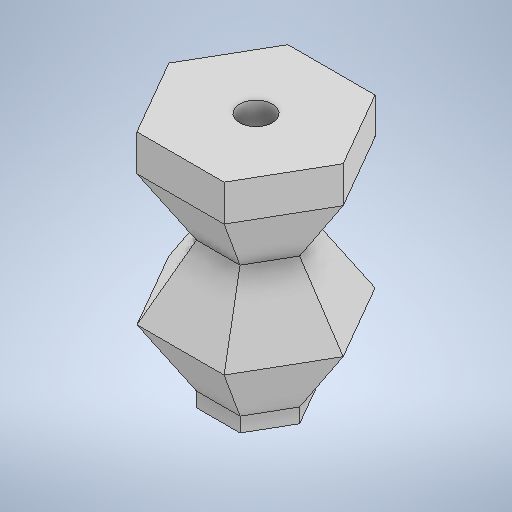
# Autodesk Inventor part: n_6
Saved by Autodesk Inventor 2025.1 (Build 291241000, 241)
## iProperties
Created: 2024-08-13
Part Number: n_6
Material: 일반
Document SubType Name: Modeling
Designer: 82103
Density: 1 g/cm^3
Appearance: 기본값
Author: 82103
Autodesk Inventor part; units mm, degrees
ref_plane "YZ Plane" through (0, 0, 0) normal (1, 0, 0) x (0, 1, 0)
ref_plane "XY Plane" through (0, 0, 0) normal (0, 0, 1) x (1, 0, 0)
sketch "스케치1" plane through (0, 0, 0) normal (0, 1, 0) x (-1, 0, 0)
  line L0 (12, 0) -> (6, -10.3923)
  line L1 (6, -10.3923) -> (-6, -10.3923)
  line L2 (-6, -10.3923) -> (-12, 0)
  line L3 (-12, 0) -> (-6, 10.3923)
  line L4 (-6, 10.3923) -> (6, 10.3923)
  line L5 (6, 10.3923) -> (12, 0)
  point P0 (0, 0)
  point P1 (0, 0)
  dimension "d0" = 24
  constraints: 12 end point, 1 coincident, 1 horizontal alignment, 13 other
  measures "d0" distance of L2.end L0.start
ref_plane "작업 평면1" through (0, 9, 0) normal (0, 1, 0) x (-1, 0, 0)
sketch "스케치2" plane through (0, 9, 0) normal (0, 1, 0) x (-1, 0, 0)
  line L0 (3, -5.1962) -> (-3, -5.1962)
  line L1 (-3, -5.1962) -> (-6, 0)
  line L2 (-6, 0) -> (-3, 5.1962)
  line L3 (-3, 5.1962) -> (3, 5.1962)
  line L4 (3, 5.1962) -> (6, 0)
  line L5 (6, 0) -> (3, -5.1962)
  point P0 (0, 0)
  point P1 (0, 0)
  dimension "d2" = 12
  constraints: 12 end point, 1 coincident, 1 horizontal alignment, 13 other
  measures "d2" distance of L1.end L4.end
loft "로프트1" add profiles "스케치2", "스케치1"
mirror "미러1" about plane through (0, 9, 0) normal (0, 1, 0) of "로프트1"
ref_plane "작업 평면2" through (0, 0, 0) normal (0, 1, 0) x (-1, 0, 0)
mirror "미러2" about plane through (0, 0, 0) normal (0, 1, 0) of "로프트1"
shell "쉘1" thickness 0.5 removed faces 0 ; own thickness 2 on faces at (-8.25, -1.5, 4.7631) (0, -1.5, 9.5263) (8.25, -1.5, 4.7631) (8.25, -1.5, -4.7631) (0, -1.5, -9.5263) (-8.25, -1.5, -4.7631) (-8.25, 16.5, -4.7631) (-8.25, 16.5, 4.7631) (0, 16.5, 9.5263) (8.25, 16.5, 4.7631) (8.25, 16.5, -4.7631) (0, 16.5, -9.5263)
sketch "스케치3" plane through (-3, -9, -5.1962) normal (0, -1, 0) x (1, 0, 0)
  line L0 (0, 0) -> (6, 0) projected
  line L1 (6, 0) -> (9, 5.1962) projected
  line L2 (9, 5.1962) -> (6, 10.3923) projected
  line L3 (6, 10.3923) -> (0, 10.3923) projected
  line L4 (0, 10.3923) -> (-3, 5.1962) projected
  line L5 (-3, 5.1962) -> (0, 0) projected
  point P0 (3, 5.1962)
extrude "돌출1" add sketch "스케치3" along normal blind 2
sketch "스케치4" plane through (-6, 18, -10.3923) normal (0, 1, 0) x (1, 0, 0)
  line L0 (0, 0) -> (12, 0) projected
  line L1 (-6, -10.3923) -> (0, 0) projected
  line L2 (0, -20.7846) -> (-6, -10.3923) projected
  line L3 (12, -20.7846) -> (0, -20.7846) projected
  line L4 (18, -10.3923) -> (12, -20.7846) projected
  line L5 (12, 0) -> (18, -10.3923) projected
  point P0 (6, -10.3923)
extrude "돌출2" add sketch "스케치4" along normal blind 5
sketch "스케치5" plane through (-6, 23, -10.3923) normal (0, 1, 0) x (1, 0, 0)
  circle A0 centre (6, -10.3923) radius 2.25
  dimension "d14" = 4.5
  constraints: 1 centre point, 1 coincident
  measures "d14" diameter of A0
extrude "돌출3" cut sketch "스케치5" against normal blind 5.5
